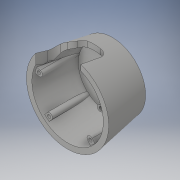
# Autodesk Inventor part: baseTop
Saved by Autodesk Inventor 2018 (Build 220112000, 112)
## iProperties
Created: 2017-04-10
Part Number: baseTop
Material: ABS Plastic
Document SubType Name: Modeling
Designer: dkt01
Density: 1.06 g/cm^3
Appearance: Light Gray
Mass: 27.4668 g
Surface Area: 144.113 cm^2
Volume: 25.9121 cm^3
Author: dkt01
Autodesk Inventor part; units mm, degrees
ref_plane "YZ Plane" through (0, 0, 0) normal (1, 0, 0) x (0, 1, 0)
ref_plane "XZ Plane" through (0, 0, 0) normal (0, 1, 0) x (-1, 0, 0)
sketch "Sketch1" plane through (0, 0, 0) normal (0, 0, 1) x (1, 0, 0)
  circle A0 centre (0, 0) radius 25
  circle A1 centre (0, 0) radius 15
  circle A2 centre (-15, 0) radius 2.5
  circle A3 centre (15, 0) radius 2.5
  circle A4 centre (0, -5) radius 4
  dimension "d1" = 30
  dimension "d0" = 50
  dimension "d2" = 5
  dimension "d5" = 360
  dimension "d8" = 8
  dimension "d9" = 5
  constraints: 4 centre point, 2 coincident, 1 horizontal alignment, 7 other
  measures "d0" diameter of A0
  measures "d2" diameter of A2
  measures "d8" diameter of A4
  measures "d9" distance of point (0, 0) A4.centre
extrude "Extrusion1" add sketch "Sketch1" along normal blind 33.7 draft 10 contours A0 | A1 A3 | A1 A3 | A3 A1 A2 | A2 A1 | A1 A2 | A4
shell "Shell1" thickness 4 removed faces 1 at (9.1327, -4.7932, 33.7)
extrude "Extrusion2" cut sketch "Sketch1" along normal blind 75 contours A1 A3 | A1 A3 | A2 A1 | A1 A2 | A4
sketch "Sketch2" plane through (0, 0, 33.7) normal (0, 0, 1) x (1, 0, 0)
  line L0 (-26.5808, 0) -> (26.5808, 0)
  line L1 (0, 0) -> (25.6165, 7.0945)
  line L2 (0, 0) -> (-25.6338, 7.0318)
  line L3 (0, 0) -> (-17.3086, -20.1729)
  line L4 (0, 0) -> (17.2381, -20.2332)
  arc A0 (-23.4325, 4.0949) -> (-22.2421, 8.4346) centre (-22.8373, 6.2647) ccw
  arc A1 (-13.6073, -19.3144) -> (-17.0225, -16.3841) centre (-15.3149, -17.8493) ccw
  arc A2 (16.8342, -16.2897) -> (13.4088, -19.208) centre (15.1215, -17.7489) ccw
  arc A3 (22.2224, 8.4892) -> (23.4234, 4.1524) centre (22.8229, 6.3208) ccw
  circle A4 centre (0, 0) radius 26.5808
  line L5 (-24.9465, 9.1764) -> (-22.2421, 8.4346)
  line L6 (-26.137, 4.8368) -> (-23.4325, 4.0949)
  line L7 (-17.0225, -16.3841) -> (-18.9541, -18.6354)
  line L8 (-15.5389, -21.5657) -> (-13.6073, -19.3144)
  line L9 (13.4088, -19.208) -> (15.4635, -21.6198)
  line L10 (16.8342, -16.2897) -> (18.8889, -18.7015)
  line L11 (22.2224, 8.4892) -> (24.924, 9.2374)
  line L12 (23.4234, 4.1524) -> (26.1251, 4.9006)
  line L13 (0, 0) -> (0, 26.5808)
  line L14 (-10, 37.1613) -> (10, 37.1613)
  line L15 (10, 37.1613) -> (10, 8.4892)
  line L16 (10, 8.4892) -> (-10, 8.4892)
  line L17 (-10, 8.4892) -> (-10, 37.1613)
  line L18 (-24, 31.6126) -> (-10, 31.6126)
  line L19 (-10, 31.6126) -> (-10, 9.4757)
  line L20 (-10, 9.4757) -> (-24, 9.4757)
  line L21 (-24, 9.4757) -> (-24, 31.6126)
  point P0 (-23.3195, 6.397)
  point P1 (-15.6405, -18.2288)
  point P2 (15.4458, -18.1295)
  point P3 (23.3048, 6.4542)
  dimension "d18" = 15.48
  dimension "d19" = 15.34
  dimension "d20" = 49.57
  dimension "d21" = 49.37
  dimension "d22" = 23.681
  dimension "d23" = 23.682
  dimension "d24" = 23.317
  dimension "d25" = 23.519
  dimension "d26" = 4.5
  dimension "d27" = 4.5
  dimension "d28" = 4.5
  dimension "d29" = 4.5
  dimension "d32" = 2.25
  dimension "d33" = 2.25
  dimension "d34" = 2.25
  dimension "d35" = 2.25
  dimension "d36" = 2.25
  dimension "d37" = 2.25
  dimension "d40" = 0.5
  dimension "d41" = 0.5
  dimension "d42" = 0.5
  dimension "d43" = 0.5
  dimension "d51" = 10
  dimension "d52" = 10
  dimension "d53" = 14
  constraints: 44 end point, 12 parallel, 9 point on line, 8 point on circle, 5 coincident, 4 centre point, 3 horizontal, 2 perpendicular, 1 vertical, 17 other
  measures "d18" angle of L0 L1
  measures "d19" angle of L0 L2
  measures "d20" angle of L4 L0
  measures "d21" angle of L0 L3
  measures "d22" distance of L1.start point (-22.837, 6.265)
  measures "d23" distance of L1.start point (22.823, 6.321)
  measures "d24" distance of point (15.122, -17.749) L1.start
  measures "d25" distance of L1.start point (-15.315, -17.849)
  measures "d26" diameter of A0
  measures "d27" diameter of A3
  measures "d28" diameter of A2
  measures "d29" diameter of A1
  measures "d32" distance between parallel lines of L3 L7
  measures "d33" distance between parallel lines of L8 L3
  measures "d34" distance between parallel lines of L4 L9
  measures "d35" distance between parallel lines of L10 L4
  measures "d36" distance between parallel lines of L1 L11
  measures "d37" distance between parallel lines of L1 L12
  measures "d40" distance of A0.centre point (-23.32, 6.397)
  measures "d41" distance of point (23.305, 6.454) point (22.823, 6.321)
  measures "d42" distance of point (15.446, -18.129) point (15.122, -17.749)
  measures "d43" distance of point (-15.315, -17.849) point (-15.64, -18.229)
  measures "d51" distance between parallel lines of L13 L17
  measures "d52" distance between parallel lines of L15 L13
  measures "d53" distance of L18.start L18.end
extrude "Extrusion4" cut sketch "Sketch2" against normal blind 20 contours L16 L17 A4 L13 | L13 A4 L15 L16 | A4 L17 L14 L15
extrude "Extrusion5" cut sketch "Sketch2" against normal blind 14 contours L17 L20 L21 A4 | A4 L21 L18 L17
fillet "Fillet1" radius 5 4 edges at (-10, 24.4648, 19.7) (-24, 12.3986, 19.7) (-10, 23.3158, 13.7) (10, 23.3158, 13.7)
ref_plane "Work Plane1" through (0, 0, 32) normal (0, 0, 1) x (1, 0, 0)
extrude "Extrusion6" add sketch "Sketch2" against normal up to next from surface at -1.7 contours A4 L2 A0 L6 | L7 A1 L3 A4 | A3 L11 A4 L1 | L1 A4 L12 A3 | L2 A4 L5 A0 | A1 L8 A4 L3 | A2 L10 A4 L4 | L4 A4 L9 A2
hole "Hole1" at (-23.3195, 6.397, 33.7) at (-15.6405, -18.2288, 33.7) at (15.4458, -18.1295, 33.7) at (23.3048, 6.4542, 33.7) direction (0, 0, -1) diameter 2.5 depth 12
body "Solid1"
